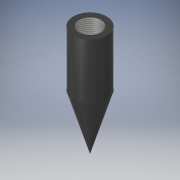
# Autodesk Inventor part: ujung tongkat
Saved by Autodesk Inventor 2019.5 (Build 235369000, 369)
## iProperties
Created: 2022-10-11
Part Number: ujung tongkat
Material: Aluminum 6061-AHC
Document SubType Name: Modeling
Designer: ASUS
Density: 2.7 g/cm^3
Appearance: Aluminum - Dark
Author: ASUS
Autodesk Inventor part; units mm, degrees
ref_plane "YZ Plane" through (0, 0, 0) normal (1, 0, 0) x (0, 1, 0)
ref_plane "XZ Plane" through (0, 0, 0) normal (0, 1, 0) x (-1, 0, 0)
ref_plane "XY Plane" through (0, 0, 0) normal (0, 0, 1) x (1, 0, 0)
sketch "Sketch2" plane through (0, 0, 0) normal (0, 0, 1) x (1, 0, 0)
  line L0 (1.453, -3.7488) -> (31.453, -3.7488)
  line L1 (1.453, -3.7488) -> (1.453, -203.7488)
  line L2 (1.453, -203.7488) -> (31.453, -103.7488)
  line L3 (31.453, -103.7488) -> (31.453, -3.7488)
  point P0 (0, 0)
  dimension "d10" = 30
  dimension "d11" = 200
  dimension "d24" = 100
  constraints: 8 end point, 2 vertical, 1 horizontal
  measures "d10" distance of L0.start L0.end
  measures "d11" distance of L0.start L1.end
  measures "d24" distance of L2.end L0.end
revolve "Revolution2" add sketch "Sketch2" angle 360 about axis through (1.453, -3.7488, 0) along (0, -1, 0)
sketch "Sketch3" plane through (1.453, -3.7488, 0) normal (0, 1, 0) x (1, 0, 0)
  circle A0 centre (0, 0) radius 30 projected
  point P0 (-1.453, 0)
  constraints: 1 coincident
hole "Hole1" at (1.453, -3.7488, 0) direction (0, -1, 0) diameter 40 depth 93.25
thread "Thread3" size "M40x3" class "6H" standard "ANSI Metric M Profile" full length
body "Solid2"
